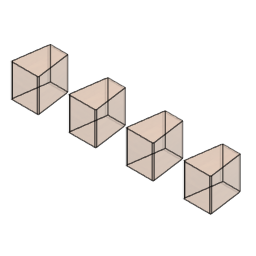
Dovetail Joint (Autodesk Fusion 360 design; units mm, degrees)
Autodesk Fusion 360 part; units mm, degrees
sketch "Contact Patch" plane through (0, 0, 0) normal (0, 0, 1) x (1, 0, 0)
  line L0 (75, -9) -> (-75, -9)
  line L1 (-75, -9) -> (-75, 9)
  line L2 (-75, 9) -> (75, 9)
  line L3 (75, 9) -> (75, -9)
  line L4 (75, -9) -> (-75, 9) construction
  line L5 (-75, -9) -> (75, 9) construction
  dimension "d3" = 150
  dimension "d4" = 18
  constraint horizontal L0
  constraint perpendicular L0 L1
  constraint parallel L0 L2
  constraint parallel L1 L3
  constraint coincident L4 origin
  constraint coincident L5 origin
  measures "d3" distance of L1.end L2.end
  measures "d4" distance of L0.end L1.end
sketch "Sketch1" plane through (0, 0, 0) normal (0, 1, 0) x (1, 0, 0) in component "Joint"
  line L0 (-55, -18) -> (-40, -18)
  line L1 (-40, -18) -> (-42.5297, 0)
  line L2 (-55, -18) -> (-52.4703, 0)
  line L3 (-75, 0) -> (75, 0)
  line L4 (-75, 0) -> (-75, -13) construction
  line L5 (-52.4703, 0) -> (-42.5297, 0)
  point P0 (-75, 0)
  dimension "d13" = 20
  dimension "d14" = 18
  dimension "d15" = 15
  dimension "d16" = 8
  constraint horizontal L0
  constraint coincident L2.end L3
  constraint coincident L1.end L3
  constraint equal L1 L2
  constraint coincident P0 L3.start
  constraint perpendicular L3 L4
  measures "d13" horizontal distance of L0.start P0
  measures "d14" distance of L0 L3
  measures "d15" distance of L0.start L0.end
  measures "d16" angle of L2 L4
extrude "Extrude1" add sketch "Sketch1" along normal blind 8.9999 and the other way blind 8.9999 makes body 1 in component "Joint"
move_face "OffsetFaces1" offset 1 1 faces at (-49.1568, -3, 0) on bodies 1 in component "Joint"
sketch "Sketch2" plane through (0, 0, 0) normal (0, 1, 0) x (1, 0, 0) in component "Joint"
  line L0 (-55, -18) -> (-40, -18)
  line L1 (-40, -18) -> (-42.6703, 1)
  line L2 (-42.6703, 1) -> (-52.3297, 1)
  line L3 (-52.3297, 1) -> (-55, -18)
  line L4 (-75, 0) -> (75, 0)
  line L5 (-52.4703, 0) -> (-42.5297, 0)
  line L6 (-52.5278, 1.0278) -> (-55.2301, -18.2)
  line L7 (-55.2301, -18.2) -> (-39.7699, -18.2)
  line L8 (-39.7699, -18.2) -> (-42.4722, 1.0278)
  line L9 (-52.6722, 0) -> (-42.3278, 0)
  dimension "d27" = 0.2
  constraint coincident L3 L5.start
  constraint coincident L4 L5.start
  constraint coincident L4 L5.end
  constraint coincident L1 L5.end
  constraint coincident L4 L9.start
  constraint coincident L6 L9.start
  constraint coincident L4 L9.end
  constraint coincident L8 L9.end
extrude "Extrude2" add sketch "Sketch2" along normal blind 9.1999 and the other way blind 9.1999 separate body contours L0 L1 L3 L4 L5 L9 | L0 L1 L3 L4 L6 L7 L8 L9 makes body 2 in component "Joint"
fillet "Fillet1" radius 0.5 2 edges at (-55, 0, 18) (-40, 0, 18) on bodies 1 in component "Joint"
pattern_linear "00000000-0000-0000-0000-000000000000" [suppressed]
component "Joint" placed x (1, 0, 0) y (0, 1, 0) z (0, 0, 1) at (0, 0, 0)
component "Joint" placed x (1, 0, 0) y (0, 1, 0) z (0, 0, 1) at (31.6667, 0, 0)
component "Joint" placed x (1, 0, 0) y (0, 1, 0) z (0, 0, 1) at (63.3333, 0, 0)
component "Joint" placed x (1, 0, 0) y (0, 1, 0) z (0, 0, 1) at (95, 0, 0)
equation "Length = 150 mm"
equation "Width = 18 mm"
equation "d3 = Length"
equation "d4 = Width"
equation "UserOffset1 = 20 mm"
equation "UserOffset2 = 20 mm"
equation "Offset1 = if(UserOffset1 < 1 mm; 5 mm; UserOffset1)"
equation "Offset2 = if(UserOffset1 < 1 mm; 5 mm; UserOffset2)"
equation "Nestled_Board_Thickness = 18 mm"
equation "Dovetail_H = Nestled_Board_Thickness"
equation "Dovetail_L = 15 mm"
equation "Dovetail_Angle = 8 deg"
equation "d13 = Offset1"
equation "d14 = Dovetail_H"
equation "d15 = Dovetail_L"
equation "d16 = Dovetail_Angle"
equation "Side_Offset1 = 0.0001 mm"
equation "Side_Offset2 = 0.0001 mm"
equation "Tenon_Width1 = ( Width / 2 ) - Side_Offset1"
equation "Tenon_Width2 = ( Width / 2 ) - Side_Offset2"
equation "d21 = Tenon_Width1"
equation "d23 = Tenon_Width2"
equation "Clearance = 0.2 mm"
equation "d27 = Clearance"
equation "d28 = Tenon_Width1 + Clearance"
equation "d30 = Tenon_Width2 + Clearance"
equation "Dovetail_QTY = 4"
equation "SpacingLength = Length - Offset1 - Offset2 - Dovetail_L"
equation "Radius = 0.5 mm"
equation "d36 = Radius"
equation "d37 = Dovetail_QTY"
equation "d39 = SpacingLength"
named bodies: "Tenon", "Mortise"
